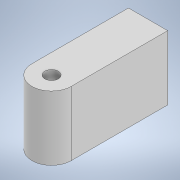
# Autodesk Inventor part: motor viber
Saved by Autodesk Inventor 2022 (Build 260153000, 153)
## iProperties
Created: 2022-05-06
Part Number: motor viber
Material: Generic
Document SubType Name: Modeling
Designer: efred
Density: 1 g/cm^3
Appearance: Default
Author: efred
Autodesk Inventor part; units mm, degrees
ref_plane "YZ Plane" through (0, 0, 0) normal (1, 0, 0) x (0, 1, 0)
ref_plane "XZ Plane" through (0, 0, 0) normal (0, 1, 0) x (-1, 0, 0)
ref_plane "XY Plane" through (0, 0, 0) normal (0, 0, 1) x (1, 0, 0)
sketch "Sketch1" plane through (0, 0, 0) normal (0, 1, 0) x (-1, 0, 0)
  circle A0 centre (0, 0) radius 1.05
  circle A1 centre (0, 0) radius 3.05
  line L0 (3.05, 0) -> (-3.05, 0) construction
  line L1 (-3.05, 0) -> (-3.05, -15)
  line L2 (-3.05, -15) -> (3.05, -15)
  line L3 (3.05, -15) -> (3.05, 0)
  dimension "d0" = 2.1
  dimension "d1" = 2
  dimension "d2" = 15
  constraints: 8 end point, 2 parallel, 2 vertical, 1 centre point, 1 coincident, 1 horizontal, 1 perpendicular, 3 other
  measures "d0" diameter of A0
  measures "d2" distance between parallel lines of L0 L2
extrude "Extrusion1" add sketch "Sketch1" along normal blind 10
body "Solid1"
